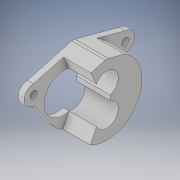
# Autodesk Inventor part: MotorFixedPositionMount
Saved by Autodesk Inventor 2017 (Build 210142000, 142)
## iProperties
Created: 2017-08-12
Part Number: MotorFixedPositionMount
Material: Generic
Document SubType Name: Modeling
Designer: User
Density: 1 g/cm^3
Appearance: Default
Author: User
Autodesk Inventor part; units mm, degrees
ref_plane "YZ Plane" through (0, 0, 0) normal (1, 0, 0) x (0, 1, 0)
ref_plane "XZ Plane" through (0, 0, 0) normal (0, 1, 0) x (-1, 0, 0)
ref_plane "XY Plane" through (0, 0, 0) normal (0, 0, 1) x (1, 0, 0)
sketch "Sketch1" plane through (0, 0, 0) normal (1, 0, 0) x (0, 1, 0)
  arc A0 (1.2261, -1.7474) -> (9.7245, 5.3822) centre (7, 0) ccw
  arc A1 (-9.7245, 5.3822) -> (-1.2261, -1.7474) centre (-7, 0) ccw
  arc A2 (9.7245, 5.3822) -> (-9.7245, 5.3822) centre (0, 8.3439) ccw
  arc A3 (-1.2261, -1.7474) -> (1.2261, -1.7474) centre (0, 8.3439) ccw
  circle A4 centre (7.0104, 24.0085) radius 1.8542
  circle A5 centre (7.0104, -23.9975) radius 1.8542
  arc A6 (12.0396, 24.0085) -> (1.9812, 24.0085) centre (7.0104, 24.0085) ccw
  arc A7 (1.9812, -23.9975) -> (12.0396, -23.9975) centre (7.0104, -23.9975) ccw
  line L0 (12.0396, 24.0085) -> (18.5, 0.0055)
  line L1 (12.0396, -23.9975) -> (18.5, 0.0055)
  line L2 (1.9812, 24.0085) -> (-13.0815, 13.087)
  line L3 (-13.0815, -13.0759) -> (1.9812, -23.9975)
  arc A8 (0.4193, 18.5008) -> (-0.4193, 18.5008) centre (0, 0.0055) ccw
  arc A9 (-13.0815, 13.087) -> (-13.0815, -13.0759) centre (0, 0.0055) ccw
  point P0 (0, 0)
  dimension "d0" = 12.065
  dimension "d1" = 7
  dimension "d2" = 12.065
  dimension "d3" = 7
  dimension "d7" = 8.3439
  dimension "d8" = 3.7084
  dimension "d11" = 3.7084
  dimension "d14" = 10.0584
  dimension "d15" = 10.0584
  dimension "d26" = 10.1655
  constraints: 18 point on circle, 10 centre point, 8 end point, 2 coincident
  measures "d0" diameter of A0
  measures "d1" distance of point (0, 0) A0.centre
  measures "d2" diameter of A1
  measures "d3" distance of A1.centre point (0, 0)
  measures "d7" distance of point (0, 0) A2.centre
  measures "d8" diameter of A4
  measures "d11" diameter of A5
  measures "d14" diameter of A6
  measures "d15" diameter of A7
  measures "d26" radius of A2
extrude "Extrusion1" add sketch "Sketch1" along normal blind 3.175
fillet "Fillet1" radius 3.175 1 edges at (1.5875, 18.5, 0.0055)
sketch "Sketch3" plane through (3.175, 0, 0) normal (1, 0, 0) x (0, 0, -1)
  arc A0 (0.8196, 18.2779) -> (-0.8307, 18.2779) centre (-0.0055, 15.212) ccw projected
  line L0 (-0.8307, 18.2779) -> (-24.0085, 12.0396) projected
  arc A1 (-24.0085, 12.0396) -> (-24.0085, 1.9812) centre (-24.0085, 7.0104) ccw projected
  line L1 (-24.0085, 1.9812) -> (-13.087, -13.0815) projected
  arc A2 (-13.087, -13.0815) -> (13.0759, -13.0815) centre (-0.0055, 0) ccw projected
  line L2 (13.0759, -13.0815) -> (23.9975, 1.9812) projected
  arc A3 (23.9975, 1.9812) -> (23.9975, 12.0396) centre (23.9975, 7.0104) ccw projected
  line L3 (23.9975, 12.0396) -> (0.8196, 18.2779) projected
  arc A4 (-5.3822, 9.7245) -> (-5.3822, -9.7245) centre (-8.3439, 0) ccw projected
  arc A5 (1.7474, 1.2261) -> (-5.3822, 9.7245) centre (0, 7) ccw projected
  arc A6 (1.7474, -1.2261) -> (1.7474, 1.2261) centre (-8.3439, 0) ccw projected
  arc A7 (-5.3822, -9.7245) -> (1.7474, -1.2261) centre (0, -7) ccw projected
  circle A8 centre (23.9975, 7.0104) radius 1.8542 projected
  circle A9 centre (-24.0085, 7.0104) radius 1.8542 projected
  line L4 (-5.3822, 9.7245) -> (-9.0442, 16.0673)
  line L5 (-5.3822, 9.7245) -> (2.0066, 9.7245) construction
  line L6 (-5.3822, -9.7245) -> (-9.0766, -16.1235)
  arc A10 (-13.087, -13.0815) -> (13.0759, -13.0815) centre (-0.0055, 0) ccw projected
  line L7 (-5.3822, -9.7245) -> (2.0066, -9.7245) construction
  arc A11 (-18.4762, 0.8213) -> (-18.4762, -0.8213) centre (0, 0) ccw
  arc A12 (16.492, -8.3701) -> (9.27, 16.0035) centre (0, 0) ccw
  line L8 (13.0759, -13.0815) -> (23.9975, 1.9812) projected
  line L9 (-5.3822, 9.7245) -> (-8.3439, 16.2557)
  line L10 (-0.8307, 18.2779) -> (-24.0085, 12.0396) projected
  line L11 (-5.3822, -9.7245) -> (-8.5881, -16.3887)
  point P0 (16.492, -8.3701)
  point P1 (-9.0073, 16.0035)
  dimension "d33" = 120
  dimension "d34" = 120
  constraints: 12 end point, 10 point on circle, 6 point on line, 2 centre point, 2 horizontal, 1 coincident, 1 equal length
  measures "d33" angle of L5 L4
  measures "d34" angle of L6 L7
extrude "Extrusion3" add sketch "Sketch3" along normal blind 14.3764 contours L3 A12 L2 A2 L11 A7 A6 A5 L9 L0 A0
body "Solid1"
